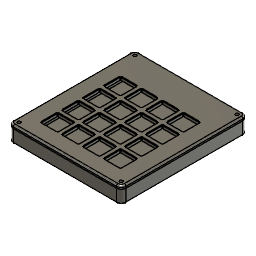
hackpad (Autodesk Fusion 360 design; units mm, degrees)
Autodesk Fusion 360 part; units mm, degrees
note: some values were not read from the file. Set by a fixed rule: which sketch regions a step uses.
(part 1 of 3)
sketch "Sketch1" plane through (0, 0, 0) normal (0, 1, 0) x (1, 0, 0)
  line L0 (0, 0) -> (87, 0)
  line L1 (87, 0) -> (87, 100)
  line L2 (87, 100) -> (0, 100)
  line L3 (0, 100) -> (0, 0)
  line L4 (-0.2, -0.2) -> (87.2, -0.2)
  line L5 (87.2, -0.2) -> (87.2, 100.2)
  line L6 (87.2, 100.2) -> (-0.2, 100.2)
  line L7 (-0.2, 100.2) -> (-0.2, -0.2)
  line L8 (-10.2, -10.2) -> (97.2, -10.2)
  line L9 (97.2, -10.2) -> (97.2, 110.2)
  line L10 (97.2, 110.2) -> (-10.2, 110.2)
  line L11 (-10.2, 110.2) -> (-10.2, -10.2)
  circle A0 centre (-5.2, 105.2) radius 1.45
  circle A1 centre (92.2, 105.2) radius 1.45
  circle A2 centre (92.2, -5.2) radius 1.45
  circle A3 centre (-5.2, -5.2) radius 1.45
  dimension "d1" = 87
  dimension "d2" = 100
  dimension "d3" = 0.2
  dimension "d4" = 10
  dimension "d5" = 2.9
  dimension "d6" = 5
  dimension "d7" = 5
  dimension "d8" = 2.9
  dimension "d9" = 5
  dimension "d10" = 5
  dimension "d11" = 2.9
  dimension "d12" = 5
  dimension "d13" = 5
  dimension "d14" = 2.9
  dimension "d15" = 5
  dimension "d16" = 5
  constraint horizontal L0
  constraint vertical L1
  constraint horizontal L2
  constraint vertical L3
  constraint coincident L0.start L3.end
  measures "d1" distance of L0.start L0.end
  measures "d2" distance of L0.start L2.end
  measures "d5" diameter of A0
  measures "d6" distance of L11 A0.centre
  measures "d7" distance of L10 A0.centre
  measures "d8" diameter of A1
  measures "d9" distance of L10 A1.centre
  measures "d10" distance of L9 A1.centre
  measures "d11" diameter of A2
  measures "d12" distance of L9 A2.centre
  measures "d13" distance of L8 A2.centre
  measures "d14" diameter of A3
  measures "d15" distance of L11 A3.centre
  measures "d16" distance of L8 A3.centre
extrude "Extrude1" add sketch "Sketch1" along normal blind 3 contours L0 L1 L2 L3 | L4 L5 L6 L7 | L8 L9 L10 L11 makes body 1
extrude "Extrude2" add sketch "Sketch1" along normal blind 13 contours L8 L9 L10 L11 bodies 1
sketch "PCB_hackpad_2026-02-28" plane through (0, 13, 0) normal (0, 1, 0) x (1, 0, 0)
  line L0 (0, 0) -> (0, 100)
  line L1 (87, 100) -> (87, 0)
  line L2 (87, 0) -> (0, 0)
  line L3 (0, 100) -> (87, 100)
  line L4 (0.5999, 71.3998) -> (0.5999, 74.5999)
  line L5 (3.3999, 71.3999) -> (3.3999, 74.5999)
  line L6 (0.5999, 51.3998) -> (0.5999, 54.5999)
  line L7 (3.3999, 51.3999) -> (3.3999, 54.5999)
  line L8 (0.5999, 31.3998) -> (0.5999, 34.5999)
  line L9 (3.3999, 31.3999) -> (3.3999, 34.5999)
  line L10 (0.5999, 11.3998) -> (0.5999, 14.5999)
  line L11 (3.3999, 11.3999) -> (3.3999, 14.5999)
  line L12 (11.3998, 3.4001) -> (14.5999, 3.4001)
  line L13 (11.3999, 0.6001) -> (14.5999, 0.6001)
  line L14 (31.3998, 3.4001) -> (34.5999, 3.4001)
  line L15 (31.3999, 0.6001) -> (34.5999, 0.6001)
  line L16 (51.3998, 3.4001) -> (54.5999, 3.4001)
  line L17 (51.3999, 0.6001) -> (54.5999, 0.6001)
  line L18 (71.3998, 3.4001) -> (74.5999, 3.4001)
  line L19 (71.3999, 0.6001) -> (74.5999, 0.6001)
  line L20 (86.2001, 14.6002) -> (86.2001, 11.4001)
  line L21 (83.4001, 14.6001) -> (83.4001, 11.4001)
  line L22 (86.2001, 34.6002) -> (86.2001, 31.4001)
  line L23 (83.4001, 34.6001) -> (83.4001, 31.4001)
  line L24 (86.2001, 54.6002) -> (86.2001, 51.4001)
  line L25 (83.4001, 54.6001) -> (83.4001, 51.4001)
  line L26 (86.2001, 74.6002) -> (86.2001, 71.4001)
  line L27 (83.4001, 74.6001) -> (83.4001, 71.4001)
  line L28 (71.3998, 86.2001) -> (74.5999, 86.2001)
  line L29 (71.3999, 83.4001) -> (74.5999, 83.4001)
  line L30 (51.3998, 86.2001) -> (54.5999, 86.2001)
  line L31 (51.3999, 83.4001) -> (54.5999, 83.4001)
  line L32 (31.3998, 86.2001) -> (34.5999, 86.2001)
  line L33 (31.3999, 83.4001) -> (34.5999, 83.4001)
  line L34 (11.3998, 86.2001) -> (14.5999, 86.2001)
  line L35 (11.3999, 83.4001) -> (14.5999, 83.4001)
  line L36 (5.3349, 80.9901) -> (20.9348, 80.9901)
  line L37 (20.9348, 65.3901) -> (5.3349, 65.3901)
  line L38 (5.3349, 65.3901) -> (5.3349, 80.9901)
  line L39 (20.9348, 80.9901) -> (20.9348, 65.3901)
  line L40 (5.3349, 45.3901) -> (5.3349, 60.9901)
  line L41 (20.9348, 45.3901) -> (5.3349, 45.3901)
  line L42 (20.9348, 60.9901) -> (20.9348, 45.3901)
  line L43 (5.3349, 60.9901) -> (20.9348, 60.9901)
  line L44 (5.3349, 40.9901) -> (20.9348, 40.9901)
  line L45 (5.3349, 25.3901) -> (5.3349, 40.9901)
  line L46 (20.9348, 25.3901) -> (5.3349, 25.3901)
  line L47 (20.9348, 40.9901) -> (20.9348, 25.3901)
  line L48 (5.3349, 20.9901) -> (20.9348, 20.9901)
  line L49 (20.9348, 5.3901) -> (5.3349, 5.3901)
  line L50 (20.9348, 20.9901) -> (20.9348, 5.3901)
  line L51 (5.3349, 5.3901) -> (5.3349, 20.9901)
  line L52 (40.9348, 20.9901) -> (40.9348, 5.3901)
  line L53 (40.9348, 5.3901) -> (25.3349, 5.3901)
  line L54 (25.3349, 20.9901) -> (40.9348, 20.9901)
  line L55 (25.3349, 5.3901) -> (25.3349, 20.9901)
  line L56 (25.3349, 25.3901) -> (25.3349, 40.9901)
  line L57 (25.3349, 40.9901) -> (40.9348, 40.9901)
  line L58 (40.9348, 25.3901) -> (25.3349, 25.3901)
  line L59 (40.9348, 40.9901) -> (40.9348, 25.3901)
  line L60 (40.9348, 60.9901) -> (40.9348, 45.3901)
  line L61 (40.9348, 45.3901) -> (25.3349, 45.3901)
  line L62 (25.3349, 60.9901) -> (40.9348, 60.9901)
  line L63 (25.3349, 45.3901) -> (25.3349, 60.9901)
  line L64 (25.3349, 80.9901) -> (40.9348, 80.9901)
  line L65 (25.3349, 65.3901) -> (25.3349, 80.9901)
  line L66 (40.9348, 80.9901) -> (40.9348, 65.3901)
  line L67 (40.9348, 65.3901) -> (25.3349, 65.3901)
  line L68 (45.3349, 5.3901) -> (45.3349, 20.9901)
  line L69 (45.3349, 20.9901) -> (60.9348, 20.9901)
  line L70 (60.9348, 20.9901) -> (60.9348, 5.3901)
  line L71 (60.9348, 5.3901) -> (45.3349, 5.3901)
  line L72 (45.3349, 40.9901) -> (60.9348, 40.9901)
  line L73 (45.3349, 25.3901) -> (45.3349, 40.9901)
  line L74 (60.9348, 40.9901) -> (60.9348, 25.3901)
  line L75 (60.9348, 25.3901) -> (45.3349, 25.3901)
  line L76 (45.3349, 45.3901) -> (45.3349, 60.9901)
  line L77 (60.9348, 60.9901) -> (60.9348, 45.3901)
  line L78 (60.9348, 45.3901) -> (45.3349, 45.3901)
  line L79 (45.3349, 60.9901) -> (60.9348, 60.9901)
  line L80 (45.3349, 65.3901) -> (45.3349, 80.9901)
  line L81 (45.3349, 80.9901) -> (60.9348, 80.9901)
  line L82 (60.9348, 65.3901) -> (45.3349, 65.3901)
  line L83 (60.9348, 80.9901) -> (60.9348, 65.3901)
  line L84 (65.3349, 5.3901) -> (65.3349, 20.9901)
  line L85 (80.9348, 5.3901) -> (65.3349, 5.3901)
  line L86 (80.9348, 20.9901) -> (80.9348, 5.3901)
  line L87 (65.3349, 20.9901) -> (80.9348, 20.9901)
  line L88 (80.9348, 25.3901) -> (65.3349, 25.3901)
  line L89 (65.3349, 40.9901) -> (80.9348, 40.9901)
  line L90 (65.3349, 25.3901) -> (65.3349, 40.9901)
  line L91 (80.9348, 40.9901) -> (80.9348, 25.3901)
  line L92 (80.9348, 45.3901) -> (65.3349, 45.3901)
  line L93 (80.9348, 60.9901) -> (80.9348, 45.3901)
  line L94 (65.3349, 60.9901) -> (80.9348, 60.9901)
  line L95 (65.3349, 45.3901) -> (65.3349, 60.9901)
  line L96 (80.9348, 65.3901) -> (65.3349, 65.3901)
  line L97 (65.3349, 65.3901) -> (65.3349, 80.9901)
  line L98 (80.9348, 80.9901) -> (80.9348, 65.3901)
  line L99 (65.3349, 80.9901) -> (80.9348, 80.9901)
  circle A0 centre (1.9997, 72.9997) radius 0.9919
  circle A1 centre (1.9997, 52.9997) radius 0.9919
  circle A2 centre (1.9997, 32.9997) radius 0.9919
  circle A3 centre (1.9997, 12.9997) radius 0.9919
  circle A4 centre (13, 2.0003) radius 0.9919
  circle A5 centre (33, 2.0003) radius 0.9919
  circle A6 centre (53, 2.0003) radius 0.9919
  circle A7 centre (73, 2.0003) radius 0.9919
  circle A8 centre (84.8004, 13) radius 0.9919
  circle A9 centre (84.8004, 33) radius 0.9919
  circle A10 centre (84.8004, 53) radius 0.9919
  circle A11 centre (84.8004, 73) radius 0.9919
  circle A12 centre (73, 84.8004) radius 0.9919
  circle A13 centre (53, 84.8004) radius 0.9919
  circle A14 centre (33, 84.8004) radius 0.9919
  circle A15 centre (13, 84.8004) radius 0.9919
  line L100 (21.984, 71.555) -> (24.016, 71.555)
  line L101 (24.0569, 70.984) -> (24.0569, 74.984)
  line L102 (21.857, 70.984) -> (24.0569, 70.984)
  line L103 (24.0569, 74.984) -> (21.857, 74.984)
  line L104 (21.857, 74.984) -> (21.857, 70.984)
  line L105 (21.984, 51.555) -> (24.016, 51.555)
  line L106 (21.857, 54.984) -> (21.857, 50.984)
  line L107 (21.857, 50.984) -> (24.0569, 50.984)
  line L108 (24.0569, 50.984) -> (24.0569, 54.984)
  line L109 (24.0569, 54.984) -> (21.857, 54.984)
  line L110 (21.984, 31.555) -> (24.016, 31.555)
  line L111 (24.0569, 30.984) -> (24.0569, 34.984)
  line L112 (24.0569, 34.984) -> (21.857, 34.984)
  line L113 (21.857, 34.984) -> (21.857, 30.984)
  line L114 (21.857, 30.984) -> (24.0569, 30.984)
  line L115 (21.984, 11.555) -> (24.016, 11.555)
  line L116 (24.0569, 14.984) -> (21.857, 14.984)
  line L117 (24.0569, 10.984) -> (24.0569, 14.984)
  line L118 (21.857, 14.984) -> (21.857, 10.984)
  line L119 (21.857, 10.984) -> (24.0569, 10.984)
  line L120 (41.984, 11.555) -> (44.016, 11.555)
  line L121 (44.0569, 10.984) -> (44.0569, 14.984)
  line L122 (41.857, 10.984) -> (44.0569, 10.984)
  line L123 (41.857, 14.984) -> (41.857, 10.984)
  line L124 (44.0569, 14.984) -> (41.857, 14.984)
  line L125 (41.984, 31.555) -> (44.016, 31.555)
  line L126 (41.857, 34.984) -> (41.857, 30.984)
  line L127 (41.857, 30.984) -> (44.0569, 30.984)
  line L128 (44.0569, 34.984) -> (41.857, 34.984)
  line L129 (44.0569, 30.984) -> (44.0569, 34.984)
  line L130 (41.984, 51.555) -> (44.016, 51.555)
  line L131 (41.857, 50.984) -> (44.0569, 50.984)
  line L132 (44.0569, 54.984) -> (41.857, 54.984)
  line L133 (44.0569, 50.984) -> (44.0569, 54.984)
  line L134 (41.857, 54.984) -> (41.857, 50.984)
  line L135 (41.984, 71.555) -> (44.016, 71.555)
  line L136 (41.857, 70.984) -> (44.0569, 70.984)
  line L137 (41.857, 74.984) -> (41.857, 70.984)
  line L138 (44.0569, 74.984) -> (41.857, 74.984)
  line L139 (44.0569, 70.984) -> (44.0569, 74.984)
  line L140 (61.984, 11.555) -> (64.016, 11.555)
  line L141 (64.0569, 14.984) -> (61.857, 14.984)
  line L142 (61.857, 10.984) -> (64.0569, 10.984)
  line L143 (64.0569, 10.984) -> (64.0569, 14.984)
  line L144 (61.857, 14.984) -> (61.857, 10.984)
  line L145 (61.984, 31.555) -> (64.016, 31.555)
  line L146 (64.0569, 34.984) -> (61.857, 34.984)
  line L147 (61.857, 30.984) -> (64.0569, 30.984)
  line L148 (61.857, 34.984) -> (61.857, 30.984)
  line L149 (64.0569, 30.984) -> (64.0569, 34.984)
  line L150 (61.984, 51.555) -> (64.016, 51.555)
  line L151 (64.0569, 50.984) -> (64.0569, 54.984)
  line L152 (61.857, 54.984) -> (61.857, 50.984)
  line L153 (64.0569, 54.984) -> (61.857, 54.984)
  line L154 (61.857, 50.984) -> (64.0569, 50.984)
  line L155 (61.984, 71.555) -> (64.016, 71.555)
  line L156 (64.0569, 70.984) -> (64.0569, 74.984)
  line L157 (61.857, 70.984) -> (64.0569, 70.984)
  line L158 (64.0569, 74.984) -> (61.857, 74.984)
  line L159 (61.857, 74.984) -> (61.857, 70.984)
  line L160 (82.984, 21.555) -> (85.016, 21.555)
  line L161 (82.857, 24.984) -> (82.857, 20.984)
  line L162 (85.0569, 24.984) -> (82.857, 24.984)
  line L163 (82.857, 20.984) -> (85.0569, 20.984)
  line L164 (85.0569, 20.984) -> (85.0569, 24.984)
  line L165 (82.984, 41.555) -> (85.016, 41.555)
  line L166 (85.0569, 40.984) -> (85.0569, 44.984)
  line L167 (82.857, 44.984) -> (82.857, 40.984)
  line L168 (82.857, 40.984) -> (85.0569, 40.984)
  line L169 (85.0569, 44.984) -> (82.857, 44.984)
  line L170 (82.984, 61.555) -> (85.016, 61.555)
  line L171 (82.857, 60.984) -> (85.0569, 60.984)
  line L172 (85.0569, 60.984) -> (85.0569, 64.984)
  line L173 (85.0569, 64.984) -> (82.857, 64.984)
  line L174 (82.857, 64.984) -> (82.857, 60.984)
  line L175 (82.984, 81.555) -> (85.016, 81.555)
  line L176 (82.857, 80.984) -> (85.0569, 80.984)
  line L177 (82.857, 84.984) -> (82.857, 80.984)
  line L178 (85.0569, 84.984) -> (82.857, 84.984)
  line L179 (85.0569, 80.984) -> (85.0569, 84.984)
  line L180 (63.1201, 97.9028) -> (63.1201, 99.7012)
  line L181 (63.1201, 99.7012) -> (80.2398, 99.7012)
  line L182 (80.9002, 99.0408) -> (80.91, 99.02)
  line L183 (80.2398, 99.7012) -> (80.9002, 99.0408)
  line L184 (63.12, 95.3633) -> (63.12, 95.7281)
  line L185 (63.12, 92.8233) -> (63.12, 93.1881)
  line L186 (63.12, 90.2833) -> (63.12, 90.6481)
  line L187 (63.12, 87.7433) -> (63.12, 88.1081)
  line L188 (63.12, 85.2033) -> (63.12, 85.5681)
  line L189 (63.12, 82.6633) -> (63.12, 83.0281)
  line L190 (63.12, 78.7) -> (63.12, 80.4881)
  line L191 (80.91, 80.5003) -> (80.91, 78.7)
  line L192 (80.91, 83.0403) -> (80.91, 82.6511)
  line L193 (80.91, 85.5803) -> (80.91, 85.1911)
  line L194 (80.91, 88.1203) -> (80.91, 87.7311)
  line L195 (80.91, 90.6603) -> (80.91, 90.2711)
  line L196 (80.91, 93.2003) -> (80.91, 92.8111)
  line L197 (80.91, 95.7403) -> (80.91, 95.3511)
  line L198 (80.91, 99.02) -> (80.91, 97.8911)
  line L199 (74.5654, 81.8729) -> (68.8504, 81.8729)
  line L200 (66.8184, 99.7799) -> (66.8184, 97.1129)
  line L201 (66.8184, 97.1129) -> (68.5964, 97.1129)
  line L202 (68.5964, 99.7799) -> (66.8184, 99.7799)
  line L203 (68.5964, 97.1129) -> (68.5964, 99.7799)
  line L204 (68.5964, 93.0464) -> (68.5964, 95.7159)
  line L205 (66.8184, 95.7159) -> (66.8184, 93.0464)
  line L206 (66.8184, 93.0464) -> (68.5964, 93.0464)
  line L207 (68.5964, 95.7159) -> (66.8184, 95.7159)
  line L208 (74.5654, 99.0179) -> (69.4854, 99.0179)
  line L209 (69.4854, 96.4779) -> (74.5654, 96.4779)
  line L210 (69.4854, 99.0179) -> (69.4854, 96.4779)
  line L211 (74.5654, 96.4779) -> (74.5654, 99.0179)
  line L212 (77.2324, 93.0464) -> (77.2324, 95.7159)
  line L213 (75.4544, 95.7159) -> (75.4544, 93.0464)
  line L214 (77.2324, 95.7159) -> (75.4544, 95.7159)
  line L215 (75.4544, 93.0464) -> (77.2324, 93.0464)
  line L216 (77.2324, 99.7799) -> (75.4544, 99.7799)
  line L217 (75.4544, 97.1129) -> (77.2324, 97.1129)
  line L218 (77.2324, 97.1129) -> (77.2324, 99.7799)
  line L219 (75.4544, 99.7799) -> (75.4544, 97.1129)
  line L220 (76.5212, 93.7677) -> (76.5212, 101.121)
  line L221 (67.522, 93.7677) -> (76.5212, 93.7677)
  line L222 (67.522, 101.121) -> (67.522, 93.7677)
  line L223 (76.5161, 101.121) -> (67.522, 101.121)
  circle A16 centre (23, 69) radius 0.4143
  circle A17 centre (23, 69) radius 0.725
  circle A18 centre (23, 77) radius 0.4143
  circle A19 centre (23, 77) radius 0.725
  circle A20 centre (23, 49) radius 0.4143
  circle A21 centre (23, 49) radius 0.725
  circle A22 centre (23, 57) radius 0.4143
  circle A23 centre (23, 57) radius 0.725
  circle A24 centre (23, 29) radius 0.4143
  circle A25 centre (23, 29) radius 0.725
  circle A26 centre (23, 37) radius 0.4143
  circle A27 centre (23, 37) radius 0.725
  circle A28 centre (23, 9) radius 0.4143
  circle A29 centre (23, 9) radius 0.725
  circle A30 centre (23, 17) radius 0.4143
  circle A31 centre (23, 17) radius 0.725
  circle A32 centre (43, 9) radius 0.4143
  circle A33 centre (43, 9) radius 0.725
  circle A34 centre (43, 17) radius 0.4143
  circle A35 centre (43, 17) radius 0.725
  circle A36 centre (43, 29) radius 0.4143
  circle A37 centre (43, 29) radius 0.725
  circle A38 centre (43, 37) radius 0.4143
  circle A39 centre (43, 37) radius 0.725
  circle A40 centre (43, 49) radius 0.4143
  circle A41 centre (43, 49) radius 0.725
  circle A42 centre (43, 57) radius 0.4143
  circle A43 centre (43, 57) radius 0.725
  circle A44 centre (43, 69) radius 0.4143
  circle A45 centre (43, 69) radius 0.725
  circle A46 centre (43, 77) radius 0.4143
  circle A47 centre (43, 77) radius 0.725
  circle A48 centre (63, 9) radius 0.4143
  circle A49 centre (63, 9) radius 0.725
  circle A50 centre (63, 17) radius 0.4143
  circle A51 centre (63, 17) radius 0.725
  circle A52 centre (63, 29) radius 0.4143
  circle A53 centre (63, 29) radius 0.725
  circle A54 centre (63, 37) radius 0.4143
  circle A55 centre (63, 37) radius 0.725
  circle A56 centre (63, 49) radius 0.4143
  circle A57 centre (63, 49) radius 0.725
  circle A58 centre (63, 57) radius 0.4143
  circle A59 centre (63, 57) radius 0.725
  circle A60 centre (63, 69) radius 0.4143
  circle A61 centre (63, 69) radius 0.725
  circle A62 centre (63, 77) radius 0.4143
  circle A63 centre (63, 77) radius 0.725
  circle A64 centre (84, 19) radius 0.4143
  circle A65 centre (84, 19) radius 0.725
  circle A66 centre (84, 27) radius 0.4143
  circle A67 centre (84, 27) radius 0.725
  circle A68 centre (84, 39) radius 0.4143
  circle A69 centre (84, 39) radius 0.725
  circle A70 centre (84, 47) radius 0.4143
  circle A71 centre (84, 47) radius 0.725
  circle A72 centre (84, 59) radius 0.4143
  circle A73 centre (84, 59) radius 0.725
  circle A74 centre (84, 67) radius 0.4143
  circle A75 centre (84, 67) radius 0.725
  circle A76 centre (84, 79) radius 0.4143
  circle A77 centre (84, 79) radius 0.725
  circle A78 centre (84, 87) radius 0.4143
  circle A79 centre (84, 87) radius 0.725
  circle A80 centre (64.467, 96.8157) radius 0.6081
  circle A81 centre (79.533, 96.8157) radius 0.6081
  circle A82 centre (79.5338, 94.2704) radius 0.6081
  circle A83 centre (79.5339, 91.7404) radius 0.6081
  circle A84 centre (79.5341, 89.2006) radius 0.6081
  circle A85 centre (79.5342, 86.6607) radius 0.6081
  circle A86 centre (79.5347, 84.1207) radius 0.6081
  circle A87 centre (79.5349, 81.5808) radius 0.6081
  circle A88 centre (64.4651, 94.2811) radius 0.6081
  circle A89 centre (64.4652, 91.7411) radius 0.6081
  circle A90 centre (64.4652, 89.2011) radius 0.6081
  circle A91 centre (64.4652, 86.6511) radius 0.6081
  circle A92 centre (64.4653, 84.1212) radius 0.6081
  circle A93 centre (64.4654, 81.5712) radius 0.6081
  circle A94 centre (23, 69) radius 0.4143
  circle A95 centre (23, 69) radius 0.725
  circle A96 centre (23, 77) radius 0.4143
  circle A97 centre (23, 77) radius 0.725
  circle A98 centre (23, 49) radius 0.4143
  circle A99 centre (23, 49) radius 0.725
  circle A100 centre (23, 57) radius 0.4143
  circle A101 centre (23, 57) radius 0.725
  circle A102 centre (23, 29) radius 0.4143
  circle A103 centre (23, 29) radius 0.725
  circle A104 centre (23, 37) radius 0.4143
  circle A105 centre (23, 37) radius 0.725
  circle A106 centre (23, 9) radius 0.4143
  circle A107 centre (23, 9) radius 0.725
  circle A108 centre (23, 17) radius 0.4143
  circle A109 centre (23, 17) radius 0.725
  circle A110 centre (43, 9) radius 0.4143
  circle A111 centre (43, 9) radius 0.725
  circle A112 centre (43, 17) radius 0.4143
  circle A113 centre (43, 17) radius 0.725
  circle A114 centre (43, 29) radius 0.4143
  circle A115 centre (43, 29) radius 0.725
  circle A116 centre (43, 37) radius 0.4143
  circle A117 centre (43, 37) radius 0.725
  circle A118 centre (43, 49) radius 0.4143
  circle A119 centre (43, 49) radius 0.725
  circle A120 centre (43, 57) radius 0.4143
  circle A121 centre (43, 57) radius 0.725
  circle A122 centre (43, 69) radius 0.4143
  circle A123 centre (43, 69) radius 0.725
  circle A124 centre (43, 77) radius 0.4143
  circle A125 centre (43, 77) radius 0.725
  circle A126 centre (63, 9) radius 0.4143
  circle A127 centre (63, 9) radius 0.725
  circle A128 centre (63, 17) radius 0.4143
  circle A129 centre (63, 17) radius 0.725
  circle A130 centre (63, 29) radius 0.4143
  circle A131 centre (63, 29) radius 0.725
  circle A132 centre (63, 37) radius 0.4143
  circle A133 centre (63, 37) radius 0.725
  circle A134 centre (63, 49) radius 0.4143
  circle A135 centre (63, 49) radius 0.725
  circle A136 centre (63, 57) radius 0.4143
  circle A137 centre (63, 57) radius 0.725
  circle A138 centre (63, 69) radius 0.4143
  circle A139 centre (63, 69) radius 0.725
  circle A140 centre (63, 77) radius 0.4143
  circle A141 centre (63, 77) radius 0.725
  circle A142 centre (84, 19) radius 0.4143
  circle A143 centre (84, 19) radius 0.725
  circle A144 centre (84, 27) radius 0.4143
  circle A145 centre (84, 27) radius 0.725
  circle A146 centre (84, 39) radius 0.4143
  circle A147 centre (84, 39) radius 0.725
  circle A148 centre (84, 47) radius 0.4143
  circle A149 centre (84, 47) radius 0.725
  circle A150 centre (84, 59) radius 0.4143
  circle A151 centre (84, 59) radius 0.725
  circle A152 centre (84, 67) radius 0.4143
  circle A153 centre (84, 67) radius 0.725
  circle A154 centre (84, 79) radius 0.4143
  circle A155 centre (84, 79) radius 0.725
  circle A156 centre (84, 87) radius 0.4143
  circle A157 centre (84, 87) radius 0.725
  circle A158 centre (73.2167, 97.5019) radius 0.5969
  circle A159 centre (73.2167, 94.9619) radius 0.5969
  circle A160 centre (70.6767, 94.9619) radius 0.5969
  circle A161 centre (70.6767, 97.5019) radius 0.5969
  circle A162 centre (64.467, 96.8157) radius 0.6081
  circle A163 centre (79.533, 96.8157) radius 0.6081
  circle A164 centre (79.5338, 94.2704) radius 0.6081
  circle A165 centre (79.5339, 91.7404) radius 0.6081
  circle A166 centre (79.5341, 89.2006) radius 0.6081
  circle A167 centre (79.5342, 86.6607) radius 0.6081
  circle A168 centre (79.5347, 84.1207) radius 0.6081
  circle A169 centre (79.5349, 81.5808) radius 0.6081
  circle A170 centre (64.4651, 94.2811) radius 0.6081
  circle A171 centre (64.4652, 91.7411) radius 0.6081
  circle A172 centre (64.4652, 89.2011) radius 0.6081
  circle A173 centre (64.4652, 86.6511) radius 0.6081
  circle A174 centre (64.4653, 84.1212) radius 0.6081
  circle A175 centre (64.4654, 81.5712) radius 0.6081
  circle A176 centre (23, 69) radius 0.4
  circle A177 centre (23, 69) radius 0.7
  circle A178 centre (23, 77) radius 0.4
  circle A179 centre (23, 77) radius 0.7
  circle A180 centre (23, 49) radius 0.4
  circle A181 centre (23, 49) radius 0.7
  circle A182 centre (23, 57) radius 0.4
  circle A183 centre (23, 57) radius 0.7
  circle A184 centre (23, 29) radius 0.4
  circle A185 centre (23, 29) radius 0.7
  circle A186 centre (23, 37) radius 0.4
  circle A187 centre (23, 37) radius 0.7
  circle A188 centre (23, 9) radius 0.4
  circle A189 centre (23, 9) radius 0.7
  circle A190 centre (23, 17) radius 0.4
  circle A191 centre (23, 17) radius 0.7
  circle A192 centre (43, 9) radius 0.4
  circle A193 centre (43, 9) radius 0.7
  circle A194 centre (43, 17) radius 0.4
  circle A195 centre (43, 17) radius 0.7
  circle A196 centre (43, 29) radius 0.4
  circle A197 centre (43, 29) radius 0.7
  circle A198 centre (43, 37) radius 0.4
  circle A199 centre (43, 37) radius 0.7
  circle A200 centre (43, 49) radius 0.4
  circle A201 centre (43, 49) radius 0.7
  circle A202 centre (43, 57) radius 0.4
  circle A203 centre (43, 57) radius 0.7
  circle A204 centre (43, 69) radius 0.4
  circle A205 centre (43, 69) radius 0.7
  circle A206 centre (43, 77) radius 0.4
  circle A207 centre (43, 77) radius 0.7
  circle A208 centre (63, 9) radius 0.4
  circle A209 centre (63, 9) radius 0.7
  circle A210 centre (63, 17) radius 0.4
  circle A211 centre (63, 17) radius 0.7
  circle A212 centre (63, 29) radius 0.4
  circle A213 centre (63, 29) radius 0.7
  circle A214 centre (63, 37) radius 0.4
  circle A215 centre (63, 37) radius 0.7
  circle A216 centre (63, 49) radius 0.4
  circle A217 centre (63, 49) radius 0.7
  circle A218 centre (63, 57) radius 0.4
  circle A219 centre (63, 57) radius 0.7
  circle A220 centre (63, 69) radius 0.4
  circle A221 centre (63, 69) radius 0.7
  circle A222 centre (63, 77) radius 0.4
  circle A223 centre (63, 77) radius 0.7
  circle A224 centre (84, 19) radius 0.4
  circle A225 centre (84, 19) radius 0.7
  circle A226 centre (84, 27) radius 0.4
  circle A227 centre (84, 27) radius 0.7
  circle A228 centre (84, 39) radius 0.4
  circle A229 centre (84, 39) radius 0.7
  circle A230 centre (84, 47) radius 0.4
  circle A231 centre (84, 47) radius 0.7
  circle A232 centre (84, 59) radius 0.4
  circle A233 centre (84, 59) radius 0.7
  circle A234 centre (84, 67) radius 0.4
  circle A235 centre (84, 67) radius 0.7
  circle A236 centre (84, 79) radius 0.4
  circle A237 centre (84, 79) radius 0.7
  circle A238 centre (84, 87) radius 0.4
  circle A239 centre (84, 87) radius 0.7
  circle A240 centre (64.467, 96.8157) radius 0.5994
  circle A241 centre (79.533, 96.8157) radius 0.5994
  circle A242 centre (79.5338, 94.2704) radius 0.5994
  circle A243 centre (79.5339, 91.7404) radius 0.5994
  circle A244 centre (79.5341, 89.2006) radius 0.5994
  circle A245 centre (79.5342, 86.6607) radius 0.5994
  circle A246 centre (79.5347, 84.1207) radius 0.5994
  circle A247 centre (79.5349, 81.5808) radius 0.5994
  circle A248 centre (64.4651, 94.2811) radius 0.5994
  circle A249 centre (64.4652, 91.7411) radius 0.5994
  circle A250 centre (64.4652, 89.2011) radius 0.5994
  circle A251 centre (64.4652, 86.6511) radius 0.5994
  circle A252 centre (64.4653, 84.1212) radius 0.5994
  circle A253 centre (64.4654, 81.5712) radius 0.5994
  circle A254 centre (2.7501, 82.0094) radius 0.305
  circle A255 centre (4.1397, 72.1394) radius 0.305
  circle A256 centre (55.3625, 4.8512) radius 0.305
  circle A257 centre (83.4765, 37.5893) radius 0.305
  circle A258 centre (84.9014, 37.0879) radius 0.305
  circle A259 centre (85.5502, 48.3719) radius 0.305
  circle A260 centre (1.2499, 56.5799) radius 0.305
  circle A261 centre (1.2629, 36.6652) radius 0.305
  circle A262 centre (1.2629, 17.0602) radius 0.305
  circle A263 centre (15.4999, 3.6609) radius 0.305
  circle A264 centre (82.4298, 9.7066) radius 0.305
  circle A265 centre (81.87, 25.6347) radius 0.305
  circle A266 centre (85.5502, 29.0599) radius 0.305
  circle A267 centre (76.9604, 65.003) radius 0.305
  circle A268 centre (84.3142, 65.0886) radius 0.305
  circle A269 centre (55.4999, 94.2799) radius 0.305
  circle A270 centre (71.8054, 89.6287) radius 0.305
  circle A271 centre (28.4125, 5.746) radius 0.305
  circle A272 centre (49.3993, 1.2499) radius 0.305
  circle A273 centre (17.4168, 5.746) radius 0.305
  circle A274 centre (1.59, 9.3917) radius 0.305
  circle A275 centre (6.1252, 12.2731) radius 0.305
  circle A276 centre (15.459, 4.683) radius 0.305
  circle A277 centre (36.6005, 2.4468) radius 0.305
  circle A278 centre (76.6005, 1.2499) radius 0.305
  circle A279 centre (50.1026, 3.6355) radius 0.305
  circle A280 centre (86.3874, 68.7488) radius 0.305
  circle A281 centre (84.05, 69.3995) radius 0.305
  circle A282 centre (3, 3) radius 1.6
  circle A283 centre (84.5001, 93) radius 1.6
  circle A284 centre (84, 2.4999) radius 1.6
  circle A285 centre (5, 90) radius 1.6
  line L224 (0.608, 74.7509) -> (0.5834, 74.7364)
  line L225 (0.4486, 74.5916) -> (0.4358, 74.566)
  line L226 (0.4974, 74.6618) -> (0.4794, 74.6396)
  line L227 (3.3128, 74.7836) -> (3.2852, 74.7907)
  line L228 (0.6335, 74.7637) -> (0.608, 74.7509)
  line L229 (0.4358, 74.566) -> (0.4249, 74.5397)
  line L230 (3.5749, 74.5397) -> (3.564, 74.566)
  line L231 (3.564, 74.566) -> (3.5512, 74.5916)
  line L232 (3.3399, 74.7746) -> (3.3128, 74.7836)
  line L233 (3.4621, 74.7022) -> (3.4399, 74.7201)
  line L234 (3.3918, 74.7509) -> (3.3663, 74.7637)
  line L235 (0.7995, 71.1999) -> (0.7999, 71.1999)
  line L236 (0.7999, 71.1999) -> (3.2, 71.1999)
  line L237 (0.3998, 74.3999) -> (0.3998, 71.5999)
  line L238 (3.4828, 71.317) -> (3.5023, 71.3379)
  line L239 (0.4291, 71.4493) -> (0.4412, 71.4223)
  line L240 (3.4399, 74.7201) -> (3.4164, 74.7364)
  line L241 (0.4412, 71.4223) -> (0.4554, 71.3962)
  line L242 (3.4164, 74.7364) -> (3.3918, 74.7509)
  line L243 (3.5908, 71.5149) -> (3.5959, 71.5429)
  line L244 (3.5839, 74.5126) -> (3.5749, 74.5397)
  line L245 (0.4892, 71.3477) -> (0.5087, 71.3254)
  line L246 (0.7406, 71.2043) -> (0.7701, 71.201)
  line L247 (3.5961, 74.4568) -> (3.591, 74.4849)
  line L248 (3.6002, 74.3999) -> (3.5991, 74.4284)
  line L249 (0.405, 71.5346) -> (0.4109, 71.5056)
  line L250 (3.5202, 71.3602) -> (3.5365, 71.3836)
  line L251 (0.5087, 71.3254) -> (0.5298, 71.3046)
  line L252 (3.4619, 71.2976) -> (3.4828, 71.317)
  line L253 (3.2569, 71.2039) -> (3.285, 71.209)
  line L254 (0.6015, 71.2524) -> (0.6277, 71.2387)
  line L255 (3.5365, 71.3836) -> (3.551, 71.4082)
  line L256 (0.5524, 71.2855) -> (0.5763, 71.268)
  line L257 (0.419, 71.4771) -> (0.4291, 71.4493)
  line L258 (3.3917, 71.2488) -> (3.4162, 71.2634)
  line L259 (0.5298, 71.3046) -> (0.5524, 71.2855)
  line L260 (3.3661, 71.236) -> (3.3917, 71.2488)
  line L261 (0.3996, 74.3999) -> (0.3998, 74.3999)
  line L262 (0.5763, 71.268) -> (0.6015, 71.2524)
  line L263 (0.3997, 71.5935) -> (0.4013, 71.564)
  line L264 (0.7996, 71.1999) -> (0.7995, 71.1999)
  line L265 (0.4554, 71.3962) -> (0.4714, 71.3713)
  line L266 (0.4109, 71.5056) -> (0.419, 71.4771)
  line L267 (3.5999, 74.3999) -> (3.6002, 74.3999)
  line L268 (3.5024, 74.6618) -> (3.483, 74.6827)
  line L269 (0.5834, 74.7364) -> (0.5599, 74.7201)
  line L270 (3.5204, 74.6396) -> (3.5024, 74.6618)
  line L271 (3.5959, 71.5429) -> (3.5989, 71.5713)
  line L272 (0.4007, 74.4284) -> (0.3996, 74.3999)
  line L273 (3.5512, 74.5916) -> (3.5366, 74.6161)
  line L274 (3.285, 71.209) -> (3.3127, 71.2161)
  line L275 (0.3998, 71.5999) -> (0.3997, 71.5935)
  line L276 (0.6829, 71.2173) -> (0.7115, 71.2097)
  line L277 (3.4397, 71.2797) -> (3.4619, 71.2976)
  line L278 (0.7427, 74.7958) -> (0.7146, 74.7907)
  line L279 (3.5366, 74.6161) -> (3.5204, 74.6396)
  line L280 (3.5999, 71.5999) -> (3.5999, 74.3999)
  line L281 (3.2285, 71.2009) -> (3.2569, 71.2039)
  line L282 (3.5991, 74.4284) -> (3.5961, 74.4568)
  line L283 (3.5747, 71.4601) -> (3.5837, 71.4872)
  line L284 (0.6277, 71.2387) -> (0.6549, 71.227)
  line L285 (3.4162, 71.2634) -> (3.4397, 71.2797)
  line L286 (3.483, 74.6827) -> (3.4621, 74.7022)
  line L287 (3.2, 71.1999) -> (3.2285, 71.2009)
  line L288 (0.687, 74.7836) -> (0.6599, 74.7746)
  line L289 (0.5168, 74.6827) -> (0.4974, 74.6618)
  line L290 (3.5989, 71.5713) -> (3.5999, 71.5999)
  line L291 (3.5638, 71.4337) -> (3.5747, 71.4601)
  line L292 (3.5837, 71.4872) -> (3.5908, 71.5149)
  line L293 (3.3127, 71.2161) -> (3.3398, 71.2251)
  line L294 (0.7701, 71.201) -> (0.7996, 71.1999)
  line L295 (3.3398, 71.2251) -> (3.3661, 71.236)
  line L296 (0.7115, 71.2097) -> (0.7406, 71.2043)
  line L297 (0.6549, 71.227) -> (0.6829, 71.2173)
  line L298 (3.551, 71.4082) -> (3.5638, 71.4337)
  line L299 (0.4013, 71.564) -> (0.405, 71.5346)
  line L300 (0.4714, 71.3713) -> (0.4892, 71.3477)
  line L301 (3.5023, 71.3379) -> (3.5202, 71.3602)
  line L302 (0.4794, 74.6396) -> (0.4632, 74.6161)
  line L303 (3.591, 74.4849) -> (3.5839, 74.5126)
  line L304 (3.2852, 74.7907) -> (3.2571, 74.7958)
  line L305 (3.3663, 74.7637) -> (3.3399, 74.7746)
  line L306 (3.2002, 74.7998) -> (0.7996, 74.7998)
  line L307 (3.2571, 74.7958) -> (3.2287, 74.7988)
  line L308 (3.2287, 74.7988) -> (3.2002, 74.7998)
  line L309 (0.5599, 74.7201) -> (0.5377, 74.7022)
  line L310 (0.4037, 74.4568) -> (0.4007, 74.4284)
  line L311 (0.6599, 74.7746) -> (0.6335, 74.7637)
  line L312 (0.7711, 74.7988) -> (0.7427, 74.7958)
  line L313 (0.4159, 74.5126) -> (0.4088, 74.4849)
  line L314 (0.4088, 74.4849) -> (0.4037, 74.4568)
  line L315 (0.4249, 74.5397) -> (0.4159, 74.5126)
  line L316 (0.4632, 74.6161) -> (0.4486, 74.5916)
  line L317 (0.5377, 74.7022) -> (0.5168, 74.6827)
  line L318 (0.7996, 74.7998) -> (0.7711, 74.7988)
  line L319 (0.7146, 74.7907) -> (0.687, 74.7836)
  line L320 (0.4088, 54.4849) -> (0.4037, 54.4568)
  line L321 (0.4794, 54.6396) -> (0.4632, 54.6161)
  line L322 (0.7427, 54.7958) -> (0.7146, 54.7907)
  line L323 (0.7711, 54.7988) -> (0.7427, 54.7958)
  line L324 (3.5747, 51.4601) -> (3.5837, 51.4872)
  line L325 (3.5999, 54.3999) -> (3.6002, 54.3999)
  line L326 (3.5837, 51.4872) -> (3.5908, 51.5149)
  line L327 (3.5365, 51.3836) -> (3.551, 51.4082)
  line L328 (3.5961, 54.4568) -> (3.591, 54.4849)
  line L329 (3.3918, 54.7509) -> (3.3663, 54.7637)
  line L330 (3.2002, 54.7998) -> (0.7996, 54.7998)
  line L331 (3.4399, 54.7201) -> (3.4164, 54.7364)
  line L332 (3.5204, 54.6396) -> (3.5024, 54.6618)
  line L333 (3.483, 54.6827) -> (3.4621, 54.7022)
  line L334 (3.2569, 51.2039) -> (3.285, 51.209)
  line L335 (3.3127, 51.2161) -> (3.3398, 51.2251)
  line L336 (3.4162, 51.2634) -> (3.4397, 51.2797)
  line L337 (3.5024, 54.6618) -> (3.483, 54.6827)
  line L338 (3.3398, 51.2251) -> (3.3661, 51.236)
  line L339 (3.5908, 51.5149) -> (3.5959, 51.5429)
  line L340 (0.4632, 54.6161) -> (0.4486, 54.5916)
  line L341 (3.4828, 51.317) -> (3.5023, 51.3379)
  line L342 (3.591, 54.4849) -> (3.5839, 54.5126)
  line L343 (3.2852, 54.7907) -> (3.2571, 54.7958)
  line L344 (3.5999, 51.5999) -> (3.5999, 54.3999)
  line L345 (3.285, 51.209) -> (3.3127, 51.2161)
  line L346 (0.4892, 51.3477) -> (0.5087, 51.3254)
  line L347 (0.4554, 51.3962) -> (0.4714, 51.3713)
  line L348 (0.5834, 54.7364) -> (0.5599, 54.7201)
  line L349 (3.5366, 54.6161) -> (3.5204, 54.6396)
  line L350 (0.5524, 51.2855) -> (0.5763, 51.268)
  line L351 (0.4109, 51.5056) -> (0.419, 51.4771)
  line L352 (0.4486, 54.5916) -> (0.4358, 54.566)
  line L353 (0.5377, 54.7022) -> (0.5168, 54.6827)
  line L354 (3.3399, 54.7746) -> (3.3128, 54.7836)
  line L355 (3.5959, 51.5429) -> (3.5989, 51.5713)
  line L356 (3.3661, 51.236) -> (3.3917, 51.2488)
  line L357 (3.4619, 51.2976) -> (3.4828, 51.317)
  line L358 (3.5749, 54.5397) -> (3.564, 54.566)
  line L359 (3.5638, 51.4337) -> (3.5747, 51.4601)
  line L360 (3.5989, 51.5713) -> (3.5999, 51.5999)
  line L361 (3.5991, 54.4284) -> (3.5961, 54.4568)
  line L362 (3.5202, 51.3602) -> (3.5365, 51.3836)
  line L363 (3.3663, 54.7637) -> (3.3399, 54.7746)
  line L364 (3.2287, 54.7988) -> (3.2002, 54.7998)
  line L365 (3.564, 54.566) -> (3.5512, 54.5916)
  line L366 (0.3998, 54.3999) -> (0.3998, 51.5999)
  line L367 (0.405, 51.5346) -> (0.4109, 51.5056)
  line L368 (0.7146, 54.7907) -> (0.687, 54.7836)
  line L369 (0.4974, 54.6618) -> (0.4794, 54.6396)
  line L370 (0.6015, 51.2524) -> (0.6277, 51.2387)
  line L371 (0.4291, 51.4493) -> (0.4412, 51.4223)
  line L372 (0.7995, 51.1999) -> (0.7999, 51.1999)
  line L373 (0.419, 51.4771) -> (0.4291, 51.4493)
  line L374 (0.4013, 51.564) -> (0.405, 51.5346)
  line L375 (0.3998, 51.5999) -> (0.3997, 51.5935)
  line L376 (0.608, 54.7509) -> (0.5834, 54.7364)
  line L377 (0.3997, 51.5935) -> (0.4013, 51.564)
  line L378 (3.2, 51.1999) -> (3.2285, 51.2009)
  line L379 (0.7999, 51.1999) -> (3.2, 51.1999)
  line L380 (0.4358, 54.566) -> (0.4249, 54.5397)
  line L381 (0.7996, 54.7998) -> (0.7711, 54.7988)
  line L382 (0.5763, 51.268) -> (0.6015, 51.2524)
  line L383 (0.4007, 54.4284) -> (0.3996, 54.3999)
  line L384 (3.4164, 54.7364) -> (3.3918, 54.7509)
  line L385 (0.5298, 51.3046) -> (0.5524, 51.2855)
  line L386 (0.6599, 54.7746) -> (0.6335, 54.7637)
  line L387 (0.3996, 54.3999) -> (0.3998, 54.3999)
  line L388 (0.7996, 51.1999) -> (0.7995, 51.1999)
  line L389 (0.6549, 51.227) -> (0.6829, 51.2173)
  line L390 (0.7406, 51.2043) -> (0.7701, 51.201)
  line L391 (0.4037, 54.4568) -> (0.4007, 54.4284)
  line L392 (0.7115, 51.2097) -> (0.7406, 51.2043)
  line L393 (3.3128, 54.7836) -> (3.2852, 54.7907)
  line L394 (3.5023, 51.3379) -> (3.5202, 51.3602)
  line L395 (0.4249, 54.5397) -> (0.4159, 54.5126)
  line L396 (3.2285, 51.2009) -> (3.2569, 51.2039)
  line L397 (0.5599, 54.7201) -> (0.5377, 54.7022)
  line L398 (0.5168, 54.6827) -> (0.4974, 54.6618)
  line L399 (0.687, 54.7836) -> (0.6599, 54.7746)
  line L400 (3.2571, 54.7958) -> (3.2287, 54.7988)
  line L401 (0.5087, 51.3254) -> (0.5298, 51.3046)
  line L402 (0.4412, 51.4223) -> (0.4554, 51.3962)
  line L403 (0.6335, 54.7637) -> (0.608, 54.7509)
  line L404 (0.6829, 51.2173) -> (0.7115, 51.2097)
  line L405 (0.7701, 51.201) -> (0.7996, 51.1999)
  line L406 (0.4714, 51.3713) -> (0.4892, 51.3477)
  line L407 (3.6002, 54.3999) -> (3.5991, 54.4284)
  line L408 (0.6277, 51.2387) -> (0.6549, 51.227)
  line L409 (0.4159, 54.5126) -> (0.4088, 54.4849)
  line L410 (3.5839, 54.5126) -> (3.5749, 54.5397)
  line L411 (3.4397, 51.2797) -> (3.4619, 51.2976)
  line L412 (3.3917, 51.2488) -> (3.4162, 51.2634)
  line L413 (3.4621, 54.7022) -> (3.4399, 54.7201)
  line L414 (3.5512, 54.5916) -> (3.5366, 54.6161)
  line L415 (3.551, 51.4082) -> (3.5638, 51.4337)
  line L416 (0.608, 34.7509) -> (0.5834, 34.7364)
  line L417 (0.7996, 34.7998) -> (0.7711, 34.7988)
  line L418 (0.5834, 34.7364) -> (0.5599, 34.7201)
  line L419 (0.4974, 34.6618) -> (0.4794, 34.6396)
  line L420 (0.6549, 31.227) -> (0.6829, 31.2173)
  line L421 (0.6277, 31.2387) -> (0.6549, 31.227)
  line L422 (0.4892, 31.3477) -> (0.5087, 31.3254)
  line L423 (0.4291, 31.4493) -> (0.4412, 31.4223)
  line L424 (0.5524, 31.2855) -> (0.5763, 31.268)
  line L425 (3.3398, 31.2251) -> (3.3661, 31.236)
  line L426 (3.564, 34.566) -> (3.5512, 34.5916)
  line L427 (0.7996, 31.1999) -> (0.7995, 31.1999)
  line L428 (3.3661, 31.236) -> (3.3917, 31.2488)
  line L429 (0.5298, 31.3046) -> (0.5524, 31.2855)
  line L430 (3.5999, 34.3999) -> (3.6002, 34.3999)
  line L431 (3.591, 34.4849) -> (3.5839, 34.5126)
  line L432 (0.3998, 34.3999) -> (0.3998, 31.5999)
  line L433 (3.4828, 31.317) -> (3.5023, 31.3379)
  line L434 (3.2, 31.1999) -> (3.2285, 31.2009)
  line L435 (3.5638, 31.4337) -> (3.5747, 31.4601)
  line L436 (3.3917, 31.2488) -> (3.4162, 31.2634)
  line L437 (0.3998, 31.5999) -> (0.3997, 31.5935)
  line L438 (3.5959, 31.5429) -> (3.5989, 31.5713)
  line L439 (0.405, 31.5346) -> (0.4109, 31.5056)
  line L440 (0.5087, 31.3254) -> (0.5298, 31.3046)
  line L441 (3.5747, 31.4601) -> (3.5837, 31.4872)
  line L442 (0.7115, 31.2097) -> (0.7406, 31.2043)
  line L443 (3.5366, 34.6161) -> (3.5204, 34.6396)
  line L444 (3.4164, 34.7364) -> (3.3918, 34.7509)
  line L445 (0.5168, 34.6827) -> (0.4974, 34.6618)
  line L446 (3.5024, 34.6618) -> (3.483, 34.6827)
  line L447 (0.4794, 34.6396) -> (0.4632, 34.6161)
  line L448 (0.7146, 34.7907) -> (0.687, 34.7836)
  line L449 (0.687, 34.7836) -> (0.6599, 34.7746)
  line L450 (0.6599, 34.7746) -> (0.6335, 34.7637)
  line L451 (0.7427, 34.7958) -> (0.7146, 34.7907)
  line L452 (0.5377, 34.7022) -> (0.5168, 34.6827)
  line L453 (0.7711, 34.7988) -> (0.7427, 34.7958)
  line L454 (3.5023, 31.3379) -> (3.5202, 31.3602)
  line L455 (3.2285, 31.2009) -> (3.2569, 31.2039)
  line L456 (0.4088, 34.4849) -> (0.4037, 34.4568)
  line L457 (0.4554, 31.3962) -> (0.4714, 31.3713)
  line L458 (0.4714, 31.3713) -> (0.4892, 31.3477)
  line L459 (3.5908, 31.5149) -> (3.5959, 31.5429)
  line L460 (0.6015, 31.2524) -> (0.6277, 31.2387)
  line L461 (0.4109, 31.5056) -> (0.419, 31.4771)
  line L462 (3.551, 31.4082) -> (3.5638, 31.4337)
  line L463 (0.4013, 31.564) -> (0.405, 31.5346)
  line L464 (3.5202, 31.3602) -> (3.5365, 31.3836)
  line L465 (0.6335, 34.7637) -> (0.608, 34.7509)
  line L466 (0.7701, 31.201) -> (0.7996, 31.1999)
  line L467 (0.3996, 34.3999) -> (0.3998, 34.3999)
  line L468 (3.5839, 34.5126) -> (3.5749, 34.5397)
  line L469 (0.7995, 31.1999) -> (0.7999, 31.1999)
  line L470 (3.5999, 31.5999) -> (3.5999, 34.3999)
  line L471 (0.7999, 31.1999) -> (3.2, 31.1999)
  line L472 (0.419, 31.4771) -> (0.4291, 31.4493)
  line L473 (0.4486, 34.5916) -> (0.4358, 34.566)
  line L474 (0.4632, 34.6161) -> (0.4486, 34.5916)
  line L475 (0.4358, 34.566) -> (0.4249, 34.5397)
  line L476 (3.3663, 34.7637) -> (3.3399, 34.7746)
  line L477 (3.4621, 34.7022) -> (3.4399, 34.7201)
  line L478 (3.2571, 34.7958) -> (3.2287, 34.7988)
  line L479 (3.2287, 34.7988) -> (3.2002, 34.7998)
  line L480 (0.4159, 34.5126) -> (0.4088, 34.4849)
  line L481 (3.5512, 34.5916) -> (3.5366, 34.6161)
  line L482 (3.2569, 31.2039) -> (3.285, 31.209)
  line L483 (3.4619, 31.2976) -> (3.4828, 31.317)
  line L484 (0.5763, 31.268) -> (0.6015, 31.2524)
  line L485 (0.4249, 34.5397) -> (0.4159, 34.5126)
  line L486 (3.3128, 34.7836) -> (3.2852, 34.7907)
  line L487 (3.5204, 34.6396) -> (3.5024, 34.6618)
  line L488 (3.3127, 31.2161) -> (3.3398, 31.2251)
  line L489 (3.4397, 31.2797) -> (3.4619, 31.2976)
  line L490 (3.5749, 34.5397) -> (3.564, 34.566)
  line L491 (0.5599, 34.7201) -> (0.5377, 34.7022)
  line L492 (0.4412, 31.4223) -> (0.4554, 31.3962)
  line L493 (3.4162, 31.2634) -> (3.4397, 31.2797)
  line L494 (3.5961, 34.4568) -> (3.591, 34.4849)
  line L495 (3.5991, 34.4284) -> (3.5961, 34.4568)
  line L496 (0.4037, 34.4568) -> (0.4007, 34.4284)
  line L497 (3.5365, 31.3836) -> (3.551, 31.4082)
  line L498 (3.6002, 34.3999) -> (3.5991, 34.4284)
  line L499 (3.5837, 31.4872) -> (3.5908, 31.5149)
  line L500 (0.7406, 31.2043) -> (0.7701, 31.201)
  line L501 (0.4007, 34.4284) -> (0.3996, 34.3999)
  line L502 (0.3997, 31.5935) -> (0.4013, 31.564)
  line L503 (0.6829, 31.2173) -> (0.7115, 31.2097)
  line L504 (3.285, 31.209) -> (3.3127, 31.2161)
  line L505 (3.5989, 31.5713) -> (3.5999, 31.5999)
  line L506 (3.3918, 34.7509) -> (3.3663, 34.7637)
  line L507 (3.3399, 34.7746) -> (3.3128, 34.7836)
  line L508 (3.4399, 34.7201) -> (3.4164, 34.7364)
  line L509 (3.483, 34.6827) -> (3.4621, 34.7022)
  line L510 (3.2852, 34.7907) -> (3.2571, 34.7958)
  line L511 (3.2002, 34.7998) -> (0.7996, 34.7998)
  line L512 (3.6002, 14.3999) -> (3.5991, 14.4284)
  line L513 (3.5024, 14.6618) -> (3.483, 14.6827)
  line L514 (0.4714, 11.3713) -> (0.4892, 11.3477)
  line L515 (0.7711, 14.7988) -> (0.7427, 14.7958)
  line L516 (0.4037, 14.4568) -> (0.4007, 14.4284)
  line L517 (0.3998, 11.5999) -> (0.3997, 11.5935)
  line L518 (0.7146, 14.7907) -> (0.687, 14.7836)
  line L519 (3.3128, 14.7836) -> (3.2852, 14.7907)
  line L520 (3.5747, 11.4601) -> (3.5837, 11.4872)
  line L521 (3.5837, 11.4872) -> (3.5908, 11.5149)
  line L522 (3.5638, 11.4337) -> (3.5747, 11.4601)
  line L523 (3.2569, 11.2039) -> (3.285, 11.209)
  line L524 (3.4399, 14.7201) -> (3.4164, 14.7364)
  line L525 (3.5366, 14.6161) -> (3.5204, 14.6396)
  line L526 (3.2287, 14.7988) -> (3.2002, 14.7998)
  line L527 (3.4164, 14.7364) -> (3.3918, 14.7509)
  line L528 (3.551, 11.4082) -> (3.5638, 11.4337)
  line L529 (0.5168, 14.6827) -> (0.4974, 14.6618)
  line L530 (3.285, 11.209) -> (3.3127, 11.2161)
  line L531 (3.5908, 11.5149) -> (3.5959, 11.5429)
  line L532 (3.5023, 11.3379) -> (3.5202, 11.3602)
  line L533 (3.3127, 11.2161) -> (3.3398, 11.2251)
  line L534 (3.3661, 11.236) -> (3.3917, 11.2488)
  line L535 (0.7427, 14.7958) -> (0.7146, 14.7907)
  line L536 (3.5749, 14.5397) -> (3.564, 14.566)
  line L537 (3.4828, 11.317) -> (3.5023, 11.3379)
  line L538 (0.4412, 11.4223) -> (0.4554, 11.3962)
  line L539 (0.5377, 14.7022) -> (0.5168, 14.6827)
  line L540 (0.4794, 14.6396) -> (0.4632, 14.6161)
  line L541 (0.7996, 11.1999) -> (0.7995, 11.1999)
  line L542 (0.7406, 11.2043) -> (0.7701, 11.201)
  line L543 (0.6829, 11.2173) -> (0.7115, 11.2097)
  line L544 (0.405, 11.5346) -> (0.4109, 11.5056)
  line L545 (0.5298, 11.3046) -> (0.5524, 11.2855)
  line L546 (0.7115, 11.2097) -> (0.7406, 11.2043)
  line L547 (0.6549, 11.227) -> (0.6829, 11.2173)
  line L548 (0.6015, 11.2524) -> (0.6277, 11.2387)
  line L549 (0.4249, 14.5397) -> (0.4159, 14.5126)
  line L550 (0.4554, 11.3962) -> (0.4714, 11.3713)
  line L551 (0.4291, 11.4493) -> (0.4412, 11.4223)
  line L552 (0.7996, 14.7998) -> (0.7711, 14.7988)
  line L553 (3.564, 14.566) -> (3.5512, 14.5916)
  line L554 (0.6335, 14.7637) -> (0.608, 14.7509)
  line L555 (0.5763, 11.268) -> (0.6015, 11.2524)
  line L556 (0.5524, 11.2855) -> (0.5763, 11.268)
  line L557 (3.4621, 14.7022) -> (3.4399, 14.7201)
  line L558 (0.4109, 11.5056) -> (0.419, 11.4771)
  line L559 (0.687, 14.7836) -> (0.6599, 14.7746)
  line L560 (0.4007, 14.4284) -> (0.3996, 14.3999)
  line L561 (0.4632, 14.6161) -> (0.4486, 14.5916)
  line L562 (0.4974, 14.6618) -> (0.4794, 14.6396)
  line L563 (0.5834, 14.7364) -> (0.5599, 14.7201)
  line L564 (0.419, 11.4771) -> (0.4291, 11.4493)
  line L565 (0.4159, 14.5126) -> (0.4088, 14.4849)
  line L566 (0.4892, 11.3477) -> (0.5087, 11.3254)
  line L567 (0.3997, 11.5935) -> (0.4013, 11.564)
  line L568 (0.3998, 14.3999) -> (0.3998, 11.5999)
  line L569 (3.2852, 14.7907) -> (3.2571, 14.7958)
  line L570 (0.3996, 14.3999) -> (0.3998, 14.3999)
  line L571 (3.3918, 14.7509) -> (3.3663, 14.7637)
  line L572 (0.5087, 11.3254) -> (0.5298, 11.3046)
  line L573 (0.4088, 14.4849) -> (0.4037, 14.4568)
  line L574 (0.4486, 14.5916) -> (0.4358, 14.566)
  line L575 (3.2, 11.1999) -> (3.2285, 11.2009)
  line L576 (0.608, 14.7509) -> (0.5834, 14.7364)
  line L577 (0.5599, 14.7201) -> (0.5377, 14.7022)
  line L578 (0.6277, 11.2387) -> (0.6549, 11.227)
  line L579 (0.6599, 14.7746) -> (0.6335, 14.7637)
  line L580 (0.7701, 11.201) -> (0.7996, 11.1999)
  line L581 (0.4013, 11.564) -> (0.405, 11.5346)
  line L582 (3.4162, 11.2634) -> (3.4397, 11.2797)
  line L583 (3.5961, 14.4568) -> (3.591, 14.4849)
  line L584 (3.3398, 11.2251) -> (3.3661, 11.236)
  line L585 (0.7999, 11.1999) -> (3.2, 11.1999)
  line L586 (3.5999, 11.5999) -> (3.5999, 14.3999)
  line L587 (3.483, 14.6827) -> (3.4621, 14.7022)
  line L588 (3.5999, 14.3999) -> (3.6002, 14.3999)
  line L589 (3.5959, 11.5429) -> (3.5989, 11.5713)
  line L590 (3.5365, 11.3836) -> (3.551, 11.4082)
  line L591 (3.5204, 14.6396) -> (3.5024, 14.6618)
  line L592 (3.2571, 14.7958) -> (3.2287, 14.7988)
  line L593 (3.5991, 14.4284) -> (3.5961, 14.4568)
  line L594 (3.5989, 11.5713) -> (3.5999, 11.5999)
  line L595 (3.2285, 11.2009) -> (3.2569, 11.2039)
  line L596 (3.4397, 11.2797) -> (3.4619, 11.2976)
  line L597 (0.7995, 11.1999) -> (0.7999, 11.1999)
  line L598 (3.2002, 14.7998) -> (0.7996, 14.7998)
  line L599 (3.3663, 14.7637) -> (3.3399, 14.7746)
  line L600 (3.3399, 14.7746) -> (3.3128, 14.7836)
  line L601 (3.5512, 14.5916) -> (3.5366, 14.6161)
  line L602 (3.5839, 14.5126) -> (3.5749, 14.5397)
  line L603 (3.591, 14.4849) -> (3.5839, 14.5126)
  line L604 (3.3917, 11.2488) -> (3.4162, 11.2634)
  line L605 (3.5202, 11.3602) -> (3.5365, 11.3836)
  line L606 (3.4619, 11.2976) -> (3.4828, 11.317)
  line L607 (0.4358, 14.566) -> (0.4249, 14.5397)
  line L608 (14.4284, 0.4009) -> (14.4568, 0.4039)
  line L609 (14.7958, 0.7429) -> (14.7988, 0.7713)
  line L610 (14.566, 0.436) -> (14.5916, 0.4488)
  line L611 (14.7746, 0.6601) -> (14.7836, 0.6872)
  line L612 (14.7988, 3.2289) -> (14.7958, 3.2573)
  line L613 (14.7958, 3.2573) -> (14.7907, 3.2854)
  line L614 (14.7637, 3.3665) -> (14.7509, 3.392)
  line L615 (14.7746, 3.3401) -> (14.7637, 3.3665)
  line L616 (14.7509, 3.392) -> (14.7364, 3.4166)
  line L617 (14.7364, 3.4166) -> (14.7201, 3.4401)
  line L618 (14.6618, 3.5026) -> (14.6396, 3.5206)
  line L619 (14.7998, 3.2004) -> (14.7988, 3.2289)
  line L620 (14.7201, 3.4401) -> (14.7022, 3.4623)
  line L621 (14.7022, 3.4623) -> (14.6827, 3.4832)
  line L622 (14.6827, 3.4832) -> (14.6618, 3.5026)
  line L623 (14.7907, 3.2854) -> (14.7836, 3.313)
  line L624 (14.7836, 3.313) -> (14.7746, 3.3401)
  line L625 (11.201, 3.2299) -> (11.1999, 3.2004)
  line L626 (11.1999, 0.8) -> (11.2009, 0.7715)
  line L627 (14.4568, 3.5963) -> (14.4284, 3.5993)
  line L628 (11.2039, 0.7431) -> (11.209, 0.715)
  line L629 (11.268, 3.4237) -> (11.2524, 3.3985)
  line L630 (11.2976, 0.5381) -> (11.317, 0.5172)
  line L631 (11.2161, 0.6873) -> (11.2251, 0.6602)
  line L632 (14.7907, 0.7148) -> (14.7958, 0.7429)
  line L633 (11.4601, 0.4253) -> (11.4872, 0.4163)
  line L634 (11.2173, 3.3171) -> (11.2097, 3.2885)
  line L635 (14.3999, 3.6004) -> (14.3999, 3.6002)
  line L636 (14.5916, 3.5514) -> (14.566, 3.5642)
  line L637 (11.317, 0.5172) -> (11.3379, 0.4977)
  line L638 (11.5149, 0.4092) -> (11.5429, 0.4041)
  line L639 (14.4284, 3.5993) -> (14.3999, 3.6004)
  line L640 (11.5429, 0.4041) -> (11.5713, 0.4011)
  line L641 (11.2251, 0.6602) -> (11.236, 0.6339)
  line L642 (11.5999, 0.4001) -> (14.3999, 0.4001)
  line L643 (11.2488, 0.6083) -> (11.2634, 0.5838)
  line L644 (11.2797, 0.5603) -> (11.2976, 0.5381)
  line L645 (11.3602, 0.4798) -> (11.3836, 0.4635)
  line L646 (14.3999, 0.4001) -> (14.3999, 0.3998)
  line L647 (11.5999, 3.6002) -> (11.5935, 3.6003)
  line L648 (11.4872, 0.4163) -> (11.5149, 0.4092)
  line L649 (11.2524, 3.3985) -> (11.2387, 3.3723)
  line L650 (11.236, 0.6339) -> (11.2488, 0.6083)
  line L651 (11.5056, 3.5891) -> (11.4771, 3.581)
  line L652 (14.3999, 3.6002) -> (11.5999, 3.6002)
  line L653 (11.1999, 3.2005) -> (11.1999, 3.2001)
  line L654 (11.5935, 3.6003) -> (11.564, 3.5987)
  line L655 (14.3999, 0.3998) -> (14.4284, 0.4009)
  line L656 (14.4849, 3.5912) -> (14.4568, 3.5963)
  line L657 (14.5397, 3.5751) -> (14.5126, 3.5841)
  line L658 (11.3962, 3.5446) -> (11.3713, 3.5286)
  line L659 (11.3254, 3.4913) -> (11.3046, 3.4702)
  line L660 (14.7201, 0.5601) -> (14.7364, 0.5836)
  line L661 (14.6396, 0.4796) -> (14.6618, 0.4976)
  line L662 (11.2009, 0.7715) -> (11.2039, 0.7431)
  line L663 (14.7637, 0.6337) -> (14.7746, 0.6601)
  line L664 (11.3379, 0.4977) -> (11.3602, 0.4798)
  line L665 (11.2855, 3.4476) -> (11.268, 3.4237)
  line L666 (14.7364, 0.5836) -> (14.7509, 0.6082)
  line L667 (11.1999, 3.2001) -> (11.1999, 0.8)
  line L668 (11.2043, 3.2594) -> (11.201, 3.2299)
  line L669 (14.6161, 3.5368) -> (14.5916, 3.5514)
  line L670 (11.564, 3.5987) -> (11.5346, 3.595)
  line L671 (14.6396, 3.5206) -> (14.6161, 3.5368)
  line L672 (11.3046, 3.4702) -> (11.2855, 3.4476)
  line L673 (11.5346, 3.595) -> (11.5056, 3.5891)
  line L674 (11.4223, 3.5588) -> (11.3962, 3.5446)
  line L675 (11.4337, 0.4362) -> (11.4601, 0.4253)
  line L676 (11.3713, 3.5286) -> (11.3477, 3.5108)
  line L677 (11.2634, 0.5838) -> (11.2797, 0.5603)
  line L678 (11.3836, 0.4635) -> (11.4082, 0.449)
  line L679 (11.4771, 3.581) -> (11.4493, 3.5709)
  line L680 (14.566, 3.5642) -> (14.5397, 3.5751)
  line L681 (11.227, 3.3451) -> (11.2173, 3.3171)
  line L682 (11.1999, 3.2004) -> (11.1999, 3.2005)
  line L683 (11.2387, 3.3723) -> (11.227, 3.3451)
  line L684 (11.4082, 0.449) -> (11.4337, 0.4362)